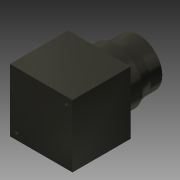
# Autodesk Inventor part: Lidar
Saved by Autodesk Inventor 2013 (Build 170138000, 138)
## iProperties
Created: 2014-12-10
Part Number: Lidar
Material: Generic
Document SubType Name: Modeling
Designer: Eyfi
Density: 1 g/cm^3
Author: Eyfi
Autodesk Inventor part; units mm, degrees
ref_plane "YZ Plane" through (0, 0, 0) normal (1, 0, 0) x (0, 1, 0)
ref_plane "XZ Plane" through (0, 0, 0) normal (0, 1, 0) x (-1, 0, 0)
ref_plane "XY Plane" through (0, 0, 0) normal (0, 0, 1) x (1, 0, 0)
sketch "Sketch1" plane through (0, 0, 0) normal (0, 1, 0) x (-1, 0, 0)
  line L0 (-24.2, -24.2) -> (24.2, -24.2)
  line L1 (24.2, -24.2) -> (24.2, 24.2)
  line L2 (24.2, 24.2) -> (-24.2, 24.2)
  line L3 (-24.2, 24.2) -> (-24.2, -24.2)
  point P0 (0, 0)
  point P1 (0, 24.2)
  point P2 (-24.2, 0)
  dimension "d0" = 48.4
  dimension "d2" = 48.4
  constraints: 8 end point, 2 midpoint, 2 parallel, 1 horizontal, 1 horizontal alignment, 1 perpendicular, 1 vertical alignment
  measures "d0" distance between parallel lines of L1 L3
  measures "d2" distance between parallel lines of L2 L0
extrude "Extrusion1" add sketch "Sketch1" along normal blind 45
sketch "Sketch2" plane through (0, 45, 0) normal (0, 1, 0) x (1, 0, 0)
  circle A0 centre (0, 0) radius 21
  dimension "d5" = 42
  constraints: 1 centre point, 1 coincident
  measures "d5" diameter of A0
extrude "Extrusion2" add sketch "Sketch2" along normal blind 12.5
sketch "Sketch3" plane through (0, 57.5, 0) normal (0, 1, 0) x (1, 0, 0)
  circle A0 centre (0, 0) radius 21 projected
  circle A1 centre (0, 0) radius 20.1325
  constraints: 1 centre point
extrude "Extrusion3" add sketch "Sketch3" along normal blind 9 contours A1
chamfer "Chamfer1" distance 2 distance2 9 1 edges at (-20.1325, 66.5, 0) measured on face at (-5.7471, 66.5, 1.5127)
sketch "Sketch4" plane through (0, 66.5, 0) normal (0, 1, 0) x (1, 0, 0)
  circle A0 centre (0, 0) radius 18.1325 projected
extrude "Extrusion4" add sketch "Sketch4" along normal blind 9
sketch "Sketch5" plane through (0, 45, 0) normal (0, 1, 0) x (1, 0, 0)
  circle A0 centre (0, 0) radius 21 projected
  line L0 (24.2, 24.2) -> (-24.2, 24.2) projected
  line L1 (-4.5, 24.2) -> (4.5, 24.2)
  line L2 (4.5, 24.2) -> (4.5, 14)
  line L3 (4.5, 14) -> (-4.5, 14)
  line L4 (-4.5, 14) -> (-4.5, 24.2)
  dimension "d16" = 9
  dimension "d18" = 4.5
  constraints: 8 end point, 2 parallel, 1 horizontal, 1 perpendicular, 1 point on line
  measures "d16" distance between parallel lines of L2 L4
  measures "d18" distance from line of A0.centre L4
extrude "Extrusion5" add sketch "Sketch5" along normal blind 20 contours L2 L3 L4 A0 | A0 L4 L0 L2 picked at (0.5035, 16.3152)
sketch "Sketch6" plane through (0, 0, 0) normal (0, -1, 0) x (1, 0, 0)
  line L0 (24.2, -24.2) -> (-24.2, -24.2) projected
  line L1 (24.2, 24.2) -> (24.2, -24.2) projected
  line L2 (-24.2, 24.2) -> (24.2, 24.2) projected
  line L3 (-24.2, -24.2) -> (-24.2, 24.2) projected
  point P0 (0, 0)
  point P1 (19.2, 19.2)
  point P2 (-19.2, -19.2)
  dimension "d21" = 5
  dimension "d22" = 5
  dimension "d23" = 5
  dimension "d24" = 5
  measures "d21" distance from line of L1 point (19.2, 19.2)
  measures "d22" distance from line of L2 point (19.2, 19.2)
  measures "d23" distance from line of L3 point (-19.2, -19.2)
  measures "d24" distance from line of L0 point (-19.2, -19.2)
hole "Hole1" at (19.2, 0, 19.2) at (-19.2, 0, -19.2) direction (0, 1, 0) diameter 2.5 depth 8 tip angle 118
sketch "Sketch7" plane through (-24.2, 0, -24.2) normal (-1, 0, 0) x (0, 0, 1)
  line L0 (38, 6) -> (44, 6)
  line L1 (44, 6) -> (44, 3)
  line L2 (44, 3) -> (38, 3)
  line L3 (38, 3) -> (38, 6)
  point P0 (24.2, 0)
  constraints: 8 end point, 2 parallel, 1 horizontal, 1 perpendicular
extrude "Extrusion6" cut sketch "Sketch7" against normal blind 5
fillet "Fillet1" radius 2 2 edges at (-21.7, 6, 13.8) (-21.7, 6, 19.8)
body "Solid1"
